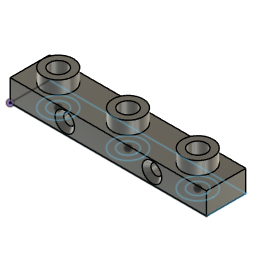
Minifix Template p2 (Autodesk Fusion 360 design; units mm, degrees)
Autodesk Fusion 360 part; units mm, degrees
sketch "Sketch1" plane through (0, 0, 0) normal (0, 0, 1) x (1, 0, 0)
  line L0 (0, 0) -> (90, 0)
  line L1 (90, 0) -> (90, 18)
  line L2 (90, 18) -> (0, 18)
  line L3 (0, 18) -> (0, 0)
  circle A0 centre (13, 9) radius 4
  circle A1 centre (45, 9) radius 4
  circle A2 centre (77, 9) radius 4
  circle A3 centre (13, 9) radius 7
  circle A4 centre (45, 9) radius 7
  circle A5 centre (77, 9) radius 7
  dimension "d1" = 9
  dimension "d2" = 9
  dimension "d3" = 9
  dimension "d4" = 45
  dimension "d5" = 32
  dimension "d6" = 32
  constraint horizontal L0
  constraint vertical L1
  constraint horizontal L2
  constraint vertical L3
  constraint coincident L0.start L3.end
  constraint concentric A0 A3
  constraint concentric A1 A4
  constraint concentric A2 A5
  measures "d1" distance of L0 A1.centre
  measures "d2" distance of L0 A2.centre
  measures "d3" distance of L0 A0.centre
  measures "d4" distance of L3 A1.centre
  measures "d5" distance of A0.centre A1.centre
  measures "d6" distance of A1.centre A2.centre
extrude "Extrude1" add sketch "Sketch1" along normal blind 10 contours L0 L1 L2 L3 | A3 | A4 | A5
extrude "Extrude2" add sketch "Sketch1" along normal blind 16 contours A3 | A4 | A5
sketch "Sketch2" plane through (0, 0, 0) normal (0, -1, 0) x (1, 0, 0)
  line L0 (0, 0) -> (90, 0)
  line L1 (90, 0) -> (90, 10)
  line L2 (90, 10) -> (0, 10)
  line L3 (0, 10) -> (0, 0)
  circle A0 centre (25, 5) radius 2.5
  circle A1 centre (65, 5) radius 2.5
  dimension "d11" = 25
  dimension "d12" = 40
  measures "d11" distance of L3 A0.centre
  measures "d12" distance of A0.centre A1.centre
extrude "Extrude3" cut sketch "Sketch2" against normal blind 18 contours A0 | A1
chamfer "Chamfer1" distance 2 angle 45 2 edges at (62.6692, 0, 5.904) (22.6692, 0, 5.904)
